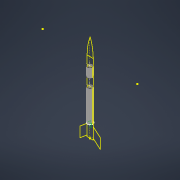
# Autodesk Inventor part: fuel tank
Saved by Autodesk Inventor 2021 (Build 250183000, 183)
## iProperties
Created: 2020-12-01
Part Number: fuel tank
Material: Stainless Steel
Document SubType Name: Modeling
Designer: henry
Density: 8 g/cm^3
Appearance: Semi-Polished
Author: henry
Autodesk Inventor part; units mm, degrees
ref_plane "YZ Plane" through (0, 0, 0) normal (1, 0, 0) x (0, 1, 0)
ref_plane "XY Plane" through (0, 0, 0) normal (0, 0, 1) x (1, 0, 0)
derived "rocket.ipt"
sketch "layout" plane through (0, 0, 0) normal (0, 0, 1) x (1, 0, 0)
  line L0 (-30, 700) -> (0, 700)
  line L1 (30, 700) -> (30, 0)
  line L2 (30, 0) -> (0, 0)
  line L3 (-30, 0) -> (-30, 700)
  line L4 (0, 0) -> (0, 870.5872) construction
  line L5 (0, 700) -> (30, 700)
  line L6 (0, 0) -> (-30, 0)
  line L7 (-25, 445.9717) -> (25, 445.9717)
  line L8 (25, 445.9717) -> (25, 135.9717)
  line L9 (25, 135.9717) -> (-25, 135.9717)
  line L10 (-25, 135.9717) -> (-25, 445.9717)
  line L11 (-25, 621.5583) -> (25, 621.5583)
  line L12 (25, 621.5583) -> (25, 531.5583)
  line L13 (25, 531.5583) -> (-25, 531.5583)
  line L14 (-25, 531.5583) -> (-25, 621.5583)
  arc A0 (0, 870.5872) -> (-30, 700) centre (470, 700) ccw
  arc A1 (30, 700) -> (0, 870.5872) centre (-470, 700) ccw
  line L15 (-30, 115) -> (-100, 56.263)
  line L16 (-100, 56.263) -> (-100, -43.737)
  line L17 (-100, -43.737) -> (-30, 15)
  line L18 (30, 115) -> (100, 56.263)
  line L19 (100, 56.263) -> (100, -43.737)
  line L20 (100, -43.737) -> (30, 15)
  line L21 (-30, 15) -> (30, 15) construction
  point P0 (0, 621.5583)
  point P1 (0, 531.5583)
  point P2 (0, 445.9717)
  point P3 (0, 135.9717)
ref_plane "ox tank bottom seam plane" through (0, 135.9717, 0) normal (0, 1, 0) x (-1, 0, 0)
sketch "ox tank wall cross section" plane through (0, 135.9717, 0) normal (0, 1, 0) x (-1, 0, 0)
  circle A0 centre (0, 0) radius 25
  circle A1 centre (0, 0) radius 27
  point P0 (-25, 0)
  dimension "d16" = 2
  constraints: 2 coincident, 1 centre point, 1 horizontal alignment, 2 other
ref_plane "tank top seam plane" through (0, 445.9717, 0) normal (0, 1, 0) x (-1, 0, 0)
extrude "oxidiser tank wall extrude" add sketch "ox tank wall cross section" along normal up to surface (310 mm away)
ref_plane "fuel tank bottom seam plane" through (0, 531.5583, 0) normal (0, 1, 0) x (-1, 0, 0)
ref_plane "fuel tank top seam plae" through (0, 621.5583, 0) normal (0, 1, 0) x (-1, 0, 0)
extrude "fuel tank wall extrude" add sketch "ox tank wall cross section" along normal up to surface (90 mm away) from surface at 395.5866 separate body
equation "\"Htank\" = 65"
